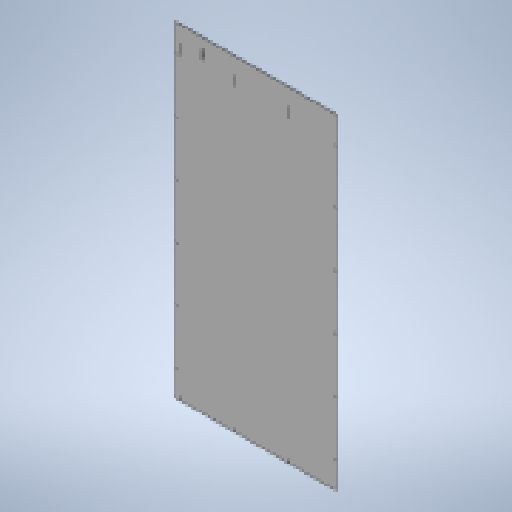
# Autodesk Inventor part: GBK 3225 shield 5
Saved by Autodesk Inventor 2026 (Build 300175000, 175)
## iProperties
Created: 2026-04-17
Part Number: GBK 3225 shield 5
Material: Steel
Document SubType Name: Sheet Metal
Designer: pokla
Stock Number: 3225
Mass: 69243.3 g
Surface Area: 44341.6 cm^2
Volume: 8820.8 cm^3
Density: 7.85 g/cm^3
Flat Pattern Width: 298 cm
Flat Pattern Length: 148 cm
Flat Pattern Area: 44104 cm^2
Sheet Metal Rule: По умолчанию_мм
Sheet Metal Width: 2980,000 мм
Sheet Metal Length: 1480,000 мм
Sheet Metal Area: 4410400,000 мм^2
Appearance: Default
Author: admin
Autodesk Inventor part; units mm, degrees
ref_plane "YZ Plane" through (0, 0, 0) normal (1, 0, 0) x (0, 1, 0)
ref_plane "XZ Plane" through (0, 0, 0) normal (0, 1, 0) x (-1, 0, 0)
ref_plane "XY Plane" through (0, 0, 0) normal (0, 0, 1) x (1, 0, 0)
sketch "Sketch1" plane through (0, 0, 0) normal (0, 0, 1) x (1, 0, 0)
  line L0 (740, -1490) -> (-740, -1490)
  line L1 (-740, -1490) -> (-740, 1490)
  line L2 (-740, 1490) -> (740, 1490)
  line L3 (740, 1490) -> (740, -1490)
  line L4 (740, -1490) -> (-740, 1490) construction
  line L5 (-740, -1490) -> (740, 1490) construction
  point P0 (0, 0)
  dimension "d0" = 1480
  dimension "d1" = 2980
  measures "d0" distance of L1.end L2.end
  measures "d1" distance of L0.end L1.end
extrude "Plate1" add sketch "Sketch1" along normal blind 4
sketch "Эскиз2" plane through (0, 0, 4) normal (0, 0, 1) x (1, 0, 0)
  line L0 (-500.3754, 1312.2758) -> (-500.3754, 1810.412) construction
  line L1 (-500.3754, 1810.412) -> (-460.7482, 1810.412) construction
  line L2 (-460.7482, 1810.412) -> (-460.7482, 1312.2758) construction
  line L3 (-460.7482, 1312.2758) -> (-500.3754, 1312.2758) construction
  line L4 (-709.6246, 1240) -> (-769.6246, 1240) projected
  line L5 (-709.6246, 1240) -> (-709.6246, 1236) projected
  line L6 (-689.2413, 1243.5) -> (-689.2413, 1340.5) projected
  line L7 (-689.2413, 1340.5) -> (-685.2413, 1340.5) projected
  line L8 (-709.6246, 743.333) -> (-769.6246, 743.333) projected
  line L9 (-709.6246, 743.333) -> (-709.6246, 739.333) projected
  line L10 (-709.6246, 246.666) -> (-769.6246, 246.666) projected
  line L11 (-709.6246, 246.666) -> (-709.6246, 242.666) projected
  line L12 (-709.6246, -250.001) -> (-769.6246, -250.001) projected
  line L13 (-709.6246, -250.001) -> (-709.6246, -254.001) projected
  line L14 (-709.6246, -746.668) -> (-769.6246, -746.668) projected
  line L15 (-709.6246, -746.668) -> (-709.6246, -750.668) projected
  line L16 (-709.6246, -1243.335) -> (-769.6246, -1243.335) projected
  line L17 (-709.6246, -1243.335) -> (-709.6246, -1247.335) projected
  line L18 (-189.3681, 1243.5) -> (-189.3681, 1340.5) projected
  line L19 (-189.3681, 1340.5) -> (-185.3681, 1340.5) projected
  line L20 (310.5051, 1243.5) -> (310.5051, 1340.5) projected
  line L21 (310.5051, 1340.5) -> (314.5051, 1340.5) projected
  line L22 (740, 1240) -> (710, 1240) projected
  line L23 (710, 1240) -> (710, 1236) projected
  line L24 (740, 743.333) -> (710, 743.333) projected
  line L25 (710, 743.333) -> (710, 739.333) projected
  line L26 (740, 246.666) -> (710, 246.666) projected
  line L27 (710, 246.666) -> (710, 242.666) projected
  line L28 (740, -250.001) -> (710, -250.001) projected
  line L29 (710, -250.001) -> (710, -254.001) projected
  line L30 (740, -746.668) -> (710, -746.668) projected
  line L31 (710, -746.668) -> (710, -750.668) projected
  line L32 (740, -1243.335) -> (710, -1243.335) projected
  line L33 (710, -1243.335) -> (710, -1247.335) projected
  line L34 (-689.2413, -1454.5) -> (-685.2413, -1454.5) projected
  line L35 (-189.3681, -1454.5) -> (-189.3681, -1514.5) projected
  line L36 (-189.3681, -1454.5) -> (-185.3681, -1454.5) projected
  line L37 (310.5051, -1454.5) -> (310.5051, -1514.5) projected
  line L38 (310.5051, -1454.5) -> (314.5051, -1454.5) projected
  line L39 (-689.2413, -1454.5) -> (-689.2413, -1514.5) projected
  point P0 (0, 0)
  constraints: 2 other
mark "Маркировка1"
equation "\"d0\" = Лист_ширина"
equation "\"d2\" = Thickness"
equation "\"BendRadius\" = Thickness"
equation "\"BendReliefWidth\" = Thickness"
equation "\"BendReliefDepth\" = 0.5 * Thickness"
equation "\"CornerReliefSize\" = 4 * Thickness"
equation "\"MinimumRemnant\" = 2 * Thickness"
equation "\"TransitionRadius\" = BendRadius"
equation "\"JacobiRadiusSize\" = BendRadius"
equation "\"GapSize\" = Thickness"
equation "\"Лист_ширина\" = 1480"
equation "\"Thickness\" = 4"
body "Solid1"
